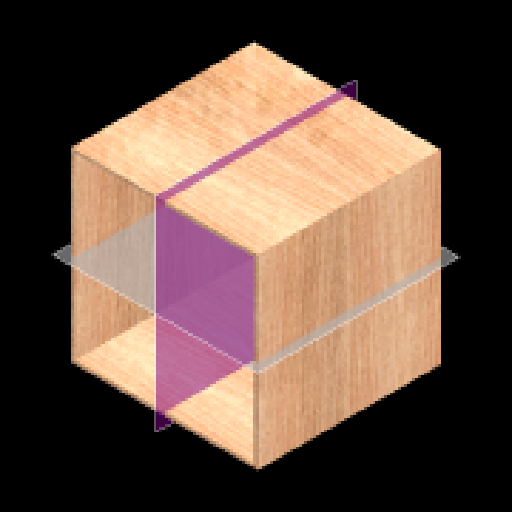
# Autodesk Inventor part: Robot Box
Saved by Autodesk Inventor 2025 (Build 290162000, 162)
## iProperties
Created: 2025-01-19
Part Number: Robot Box
Material: Wood (Birch)
Document SubType Name: Modeling
Designer: Trevor
Density: 0.55 g/cm^3
Appearance: Birch - Natural Polished
Author: Trevor
Autodesk Inventor part; units mm, degrees
ref_plane "YZ Plane" through (0, 0, 0) normal (1, 0, 0) x (0, 1, 0)
ref_plane "XZ Plane" through (0, 0, 0) normal (0, 1, 0) x (-1, 0, 0)
ref_plane "XY Plane" through (0, 0, 0) normal (0, 0, 1) x (1, 0, 0)
sketch "Sketch1" plane through (0, 0, 0) normal (0, 0, 1) x (1, 0, 0)
  line L0 (-152.4, -152.4) -> (152.4, -152.4)
  line L1 (152.4, -152.4) -> (152.4, 152.4)
  line L2 (152.4, 152.4) -> (-152.4, 152.4)
  line L3 (-152.4, 152.4) -> (-152.4, -152.4)
  line L4 (-152.4, -152.4) -> (152.4, 152.4) construction
  line L5 (152.4, -152.4) -> (-152.4, 152.4) construction
  point P0 (0, 0)
  dimension "d0" = 304.8
  dimension "d1" = 304.8
  constraints: 12 end point, 2 midpoint, 2 parallel, 1 horizontal, 1 perpendicular
  measures "d0" distance of L2.end L1.end
  measures "d1" distance of L1.end L0.end
extrude "Extrusion1" add sketch "Sketch1" along normal blind 6.35
sketch "Sketch2" plane through (152.4, -152.4, 0) normal (1, 0, 0) x (0, 0, -1)
  line L0 (-6.35, 0) -> (-6.35, 304.8) projected
  line L1 (-6.35, 304.8) -> (-311.15, 304.8)
  line L2 (-311.15, 304.8) -> (-311.15, 0)
  line L3 (-311.15, 0) -> (-6.35, 0)
  line L4 (-6.35, 0) -> (-6.35, 304.8)
  line L5 (0, 0) -> (0, 304.8) projected
  line L6 (0, 304.8) -> (-6.35, 304.8) projected
  line L7 (-6.35, 0) -> (-6.35, 304.8) projected
  line L8 (0, 0) -> (-6.35, 0) projected
  point P0 (0, 152.4)
  dimension "d4" = 304.8
  dimension "d5" = 304.8
  constraints: 8 end point, 2 parallel, 1 horizontal, 1 perpendicular
  measures "d4" distance of L3.end L2.end
  measures "d5" distance of L2.end L1.end
extrude "Extrusion2" add sketch "Sketch2" along normal blind 6.35
sketch "Sketch3" plane through (152.4, 152.4, 311.15) normal (0, 1, 0) x (1, 0, 0)
  line L0 (0, 304.8) -> (-304.8, 304.8) projected
  line L1 (0, 304.8) -> (0, 0) projected
  line L2 (0, 304.8) -> (-304.8, 304.8)
  line L3 (-304.8, 304.8) -> (-304.8, 0)
  line L4 (-304.8, 0) -> (0, 0)
  line L5 (0, 0) -> (0, 304.8)
  line L6 (-304.8, 311.15) -> (6.35, 311.15) projected
  line L7 (-304.8, 311.15) -> (-304.8, 304.8) projected
  line L8 (0, 304.8) -> (-304.8, 304.8) projected
  line L9 (0, 304.8) -> (0, 0) projected
  line L10 (0, 0) -> (6.35, 0) projected
  line L11 (6.35, 311.15) -> (6.35, 0) projected
  point P0 (-152.4, 311.15)
  dimension "d8" = 304.8
  dimension "d9" = 304.8
  constraints: 8 end point, 2 parallel, 1 horizontal, 1 perpendicular
  measures "d8" distance of L4.end L3.end
  measures "d9" distance of L3.end L2.end
extrude "Extrusion3" add sketch "Sketch3" along normal blind 6.35
sketch "Sketch4" plane through (-152.4, 152.4, 6.35) normal (-1, 0, 0) x (0, 0, 1)
  line L0 (-6.35, -304.8) -> (-6.35, 6.35) projected
  line L1 (-6.35, -304.8) -> (0, -304.8) projected
  line L2 (0, 0) -> (0, -304.8) projected
  line L3 (0, 0) -> (304.8, 0) projected
  line L4 (304.8, 0) -> (304.8, 6.35) projected
  line L5 (-6.35, 6.35) -> (304.8, 6.35) projected
  line L6 (0, 0) -> (304.8, 0)
  line L7 (304.8, 0) -> (304.8, -304.8)
  line L8 (304.8, -304.8) -> (0, -304.8)
  line L9 (0, -304.8) -> (0, 0)
  point P0 (-6.35, -152.4)
  dimension "d12" = 304.8
  dimension "d13" = 304.8
  constraints: 8 end point, 2 parallel, 1 horizontal, 1 perpendicular
  measures "d12" distance of L7.end L8.end
  measures "d13" distance of L6.end L7.end
extrude "Extrusion4" add sketch "Sketch4" along normal blind 6.35
sketch "Sketch5" plane through (152.4, -152.4, 6.35) normal (0, -1, 0) x (1, 0, 0)
  line L0 (6.35, -6.35) -> (-311.15, -6.35) projected
  line L1 (6.35, 304.8) -> (6.35, -6.35) projected
  line L2 (0, 304.8) -> (6.35, 304.8) projected
  line L3 (0, 304.8) -> (0, 0) projected
  line L4 (-304.8, 0) -> (0, 0) projected
  line L5 (-304.8, 0) -> (-304.8, 304.8) projected
  line L6 (-304.8, 304.8) -> (-311.15, 304.8) projected
  line L7 (-311.15, -6.35) -> (-311.15, 304.8) projected
  line L8 (-304.8, 0) -> (0, 0)
  line L9 (0, 0) -> (0, 304.8)
  line L10 (0, 304.8) -> (-304.8, 304.8)
  line L11 (-304.8, 304.8) -> (-304.8, 0)
  point P0 (-152.4, -6.35)
  dimension "d16" = 304.8
  dimension "d17" = 304.8
  constraints: 8 end point, 2 parallel, 1 horizontal, 1 perpendicular
  measures "d16" distance of L10.end L2.start
  measures "d17" distance of L2.start L8.end
extrude "Extrusion5" add sketch "Sketch5" along normal blind 6.35
ref_plane "Work Plane1" through (152.4, 0, 311.15) normal (0, 1, 0) x (1, 0, 0)
ref_plane "Work Plane2" through (0, 152.4, 6.35) normal (-1, 0, 0) x (0, 0, 1)
body "Solid1"
